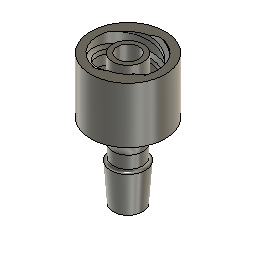
Luer Connector Female Lock (Autodesk Fusion 360 design; units mm, degrees)
Autodesk Fusion 360 part; units mm, degrees
sketch "Sketch1" plane through (0, 0, 0) normal (0, 0, 1) x (1, 0, 0)
  circle A0 centre (0, 0) radius 5
  dimension "d1" = 10
  constraint coincident A0.centre origin
  measures "d1" diameter of A0
extrude "Extrude1" add sketch "Sketch1" along normal blind 2
sketch "Sketch4" plane through (0, 0, 2) normal (0, 0, 1) x (1, 0, 0)
  circle A0 centre (0, 0) radius 2.2254
  circle A1 centre (0, 0) radius 1.45
  arc A2 (1.42, 3.207) -> (-1.1139, 3.3257) centre (0, 0) ccw
  arc A3 (2.735, 2.9382) -> (1.42, 3.207) centre (1.417, -0.159) ccw
  arc A4 (-1.1139, 3.3257) -> (-2.6284, 3.1064) centre (-1.332, -0.506) ccw
  arc A5 (-1.42, -3.207) -> (1.1139, -3.3257) centre (0, 0) ccw
  arc A6 (-2.735, -2.9382) -> (-1.42, -3.207) centre (-1.417, 0.159) ccw
  arc A7 (1.1139, -3.3257) -> (2.6284, -3.1064) centre (1.332, 0.506) ccw
  line L0 (0, 0, 0) -> (0, 0, 5.5)
  circle A8 centre (0, 0) radius 4
  circle A9 centre (0, 0) radius 5
extrude "Extrude8" add sketch "Sketch4" along normal blind 5.5 draft -1.72 contours A0 | A1
extrude "Extrude9" cut sketch "Sketch4" along normal blind 7.5 contours A1
extrude "Extrude10" add sketch "Sketch4" along normal blind 5.5 contours A9
sweep "Sweep3" add twist angle 396 profiles "Sketch4" path "Sketch4" along L0 section 1 contours A2 A3 A4 A8 | A5 A6 A7 A8
sketch "Sketch6" plane through (0, 0, 0) normal (0, 1, 0) x (1, 0, 0)
  line L0 (0, 0) -> (-2, 0)
  line L1 (-2, 0) -> (-2, 5)
  line L2 (-2, 5) -> (-2.35, 5)
  line L3 (-2.35, 5) -> (-2, 10)
  line L4 (-2, 10) -> (0, 10)
  line L5 (0, 10) -> (0, 0)
  dimension "d41" = 2
  dimension "d42" = 0.35
  constraint coincident L0.start L5.end
  constraint horizontal L0
  constraint perpendicular L0 L1
  constraint perpendicular L1 L2
  constraint perpendicular L1 L4
  constraint perpendicular L0 L5
  measures "d41" distance of L0.start L0.end
  measures "d42" distance of L1.end L2.end
revolve "Revolve1" add sketch "Sketch6" angle 360 about axis through (0, 0, 1.75) along (0, 0, 1)
fillet "Fillet1" radius 3 1 edges at (1.8647, 0.7232, 0)
sketch "Sketch7" plane through (0, 0, -10) normal (0, 0, -1) x (1, 0, 0)
  circle A0 centre (0, 0) radius 2
  circle A1 centre (0, 0) radius 1.45
  dimension "d46" = 2.9
  constraint coincident A0.centre A1.centre
  measures "d46" diameter of A1
extrude "Extrude11" cut sketch "Sketch7" against normal blind 12 contours A1
fillet "Fillet2" radius 0.3 1 edges at (-1.3519, -0.5243, -10)
fillet "Fillet3" radius 0.35 1 edges at (-1.8647, 0.7232, -5)
fillet "Fillet4" radius 1 1 edges at (-2.0748, 0.8047, 2)
